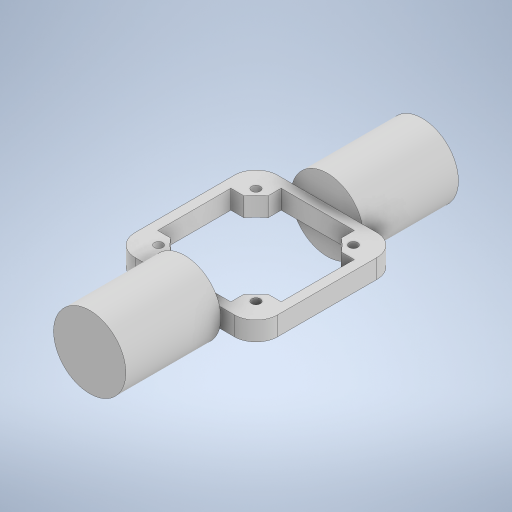
# Autodesk Inventor part: FrontPlateV2
Saved by Autodesk Inventor 2024 (Build 280153000, 153)
## iProperties
Created: 2024-02-08
Part Number: FrontPlateV2
Material: Generic
Document SubType Name: Modeling
Designer: yusuf
Density: 1 g/cm^3
Appearance: Default
Author: yusuf
Autodesk Inventor part; units mm, degrees
ref_plane "YZ Plane" through (0, 0, 0) normal (1, 0, 0) x (0, 1, 0)
ref_plane "XZ Plane" through (0, 0, 0) normal (0, 1, 0) x (-1, 0, 0)
ref_plane "XY Plane" through (0, 0, 0) normal (0, 0, 1) x (1, 0, 0)
sketch "Sketch1" plane through (0, 0, 0) normal (0, 0, 1) x (1, 0, 0)
  circle A0 centre (0, 0) radius 38
  dimension "d0" = 76
  constraints: 1 centre point, 1 coincident
  measures "d0" diameter of A0
extrude "Extrusion1" add sketch "Sketch1" along normal blind 100
sketch "Sketch2" plane through (0, 0, 0) normal (0, 0, -1) x (-1, 0, 0)
  circle A0 centre (0, 0) radius 8.75
  line L0 (0, 8.75) -> (0, 11.75)
  line L1 (0, 11.75) -> (4, 11.75)
  line L2 (4, 11.75) -> (-4, 11.75)
  line L3 (-4, 11.75) -> (-4, 7.7822)
  line L4 (4, 11.75) -> (4, 7.7822)
  dimension "d3" = 17.5
  dimension "d5" = 3
  dimension "d6" = 4
  dimension "d7" = 8
  dimension "d8" = 3.9678
  dimension "d9" = 3.9678
  constraints: 10 end point, 3 point on circle, 2 vertical, 1 centre point, 1 coincident, 1 horizontal, 1 point on line
  measures "d3" diameter of A0
  measures "d5" distance of L0.start L0.end
  measures "d6" distance of L0.end L1.end
  measures "d7" distance of L1.end L2.end
  measures "d8" distance of L2.end L3.end
  measures "d9" distance of L1.end L4.end
extrude "Extrusion2" cut sketch "Sketch2" against normal blind 90
fillet "Fillet1" radius 0.5 4 edges at (4, 9.7661, 0) (0, 11.75, 0) (-4, 9.7661, 0) (0, -8.75, 0)
fillet "Fillet2" radius 0.5 4 edges at (-4, 7.7822, 45.25) (-4.1498, 7.8731, 0.1431) (4, 7.7822, 45.25) (4.1498, 7.8731, 0.1431)
sketch "Sketch5" plane through (0, 0, 100) normal (0, 0, 1) x (1, 0, 0)
  line L0 (-75, -10) -> (75, -10)
  line L1 (75, -10) -> (75, 10)
  line L2 (75, 10) -> (-75, 10)
  line L3 (-75, 10) -> (-75, -10)
  line L4 (-75, -10) -> (75, 10) construction
  line L5 (75, -10) -> (-75, 10) construction
  point P0 (0, 0)
  dimension "d32" = 150
  dimension "d33" = 20
  constraints: 12 end point, 2 midpoint, 2 parallel, 1 horizontal, 1 perpendicular
  measures "d32" distance of L1.end L2.end
  measures "d33" distance of L0.end L1.end
extrude "Extrusion5" add sketch "Sketch5" along normal blind 150
fillet "Fillet6" radius 22.751 4 edges at (-75, 0, 250) (75, 0, 250) (75, 0, 100) (-75, 0, 100)
sketch "Sketch8" plane through (0, 0, 250) normal (0, 0, 1) x (1, 0, 0)
  circle A0 centre (0, 0) radius 38
  constraints: 1 centre point, 1 coincident
extrude "Extrusion8" add sketch "Sketch8" along normal blind 100
sketch "Sketch11" plane through (-36.6606, 10, 100) normal (0, 1, 0) x (1, 0, 0)
  line L0 (-28.3394, -140) -> (101.6606, -140)
  line L1 (101.6606, -140) -> (101.6606, -10)
  line L2 (101.6606, -10) -> (-28.3394, -10)
  line L3 (-28.3394, -10) -> (-28.3394, -140)
  line L4 (-28.3394, -140) -> (101.6606, -10) construction
  line L5 (101.6606, -140) -> (-28.3394, -10) construction
  line L6 (-38.3394, -22.751) -> (-38.3394, -127.249) projected
  line L7 (0, -150) -> (73.3212, -150) projected
  line L8 (-38.3394, -127.249) -> (-28.3394, -127.249)
  line L9 (-15.5884, -150) -> (0, -150) projected
  line L10 (-15.5884, -150) -> (-15.5884, -140)
  line L11 (-38.3394, -22.751) -> (-38.3394, -127.249) projected
  line L12 (-38.3394, -22.751) -> (-28.3394, -22.751)
  arc A0 (-15.5884, 0) -> (-38.3394, -22.751) centre (-15.5884, -22.751) ccw projected
  line L13 (-15.5884, 0) -> (-15.5884, -10)
  line L14 (88.9096, 0) -> (73.3212, 0) projected
  line L15 (88.9096, 0) -> (88.9096, -10)
  arc A1 (111.6606, -22.751) -> (88.9096, 0) centre (88.9096, -22.751) ccw projected
  line L16 (111.6606, -22.751) -> (101.6606, -22.751)
  line L17 (73.3212, -150) -> (88.9096, -150) projected
  line L18 (88.9096, -150) -> (88.9096, -140)
  line L19 (111.6606, -22.751) -> (111.6606, -127.249) projected
  line L20 (111.6606, -127.249) -> (101.6606, -127.249)
  line L21 (-28.3394, -75) -> (-28.3394, -36.5)
  line L22 (-28.3394, -75) -> (-28.3394, -113.5)
  line L23 (-28.3394, -36.5) -> (-14.5394, -36.5)
  line L24 (36.6606, -10) -> (-1.8394, -10)
  line L25 (36.6606, -10) -> (75.1606, -10)
  line L26 (-1.8394, -10) -> (-1.8394, -23.8)
  arc A2 (-1.8394, -23.8) -> (-14.5394, -36.5) centre (36.832, -75.1714) ccw
  line L27 (36.6606, -140) -> (-1.8394, -140)
  line L28 (36.6606, -140) -> (75.1606, -140)
  line L29 (101.6606, -75) -> (101.6606, -113.5)
  line L30 (101.6606, -75) -> (101.6606, -36.5)
  line L31 (36.6606, -10) -> (75.1606, -10)
  line L32 (-28.3394, -113.5) -> (-14.5394, -113.5)
  line L33 (-1.8394, -140) -> (-1.8394, -126.2)
  line L34 (75.1606, -140) -> (75.1606, -126.2)
  line L35 (101.6606, -113.5) -> (87.8606, -113.5)
  line L36 (101.6606, -36.5) -> (87.8606, -36.5)
  line L37 (75.1606, -10) -> (75.1606, -23.8)
  arc A3 (75.1606, -126.2) -> (87.8606, -113.5) centre (36.4892, -74.8286) ccw
  arc A4 (-14.5394, -113.5) -> (-1.8394, -126.2) centre (36.832, -74.8286) ccw
  arc A5 (87.8606, -36.5) -> (75.1606, -23.8) centre (36.4892, -75.1714) ccw
  point P0 (36.6606, 100)
  point P1 (36.6606, -75)
  dimension "d72" = 130
  dimension "d73" = 130
  dimension "d74" = 75
  dimension "d75" = 75
  dimension "d84" = 38.5
  dimension "d85" = 38.5
  dimension "d86" = 13.8
  dimension "d87" = 38.5
  dimension "d88" = 38.5
  dimension "d89" = 13.8
  dimension "d90" = 64.3
  dimension "d96" = 38.5
  dimension "d97" = 38.5
  dimension "d98" = 38.5
  dimension "d99" = 38.5
  dimension "d100" = 13.8
  dimension "d101" = 13.8
  dimension "d102" = 13.8
  dimension "d103" = 13.8
  dimension "d104" = 13.8
  dimension "d105" = 13.8
  dimension "d106" = 64.3
  dimension "d107" = 64.3
  dimension "d108" = 64.3
  constraints: 62 end point, 20 point on line, 8 point on circle, 6 midpoint, 5 horizontal, 5 perpendicular, 4 centre point, 4 vertical, 3 equal length
  measures "d72" distance of L1.end L2.end
  measures "d73" distance of L0.end L1.end
  measures "d74" distance from line of point (36.661, -75) L6
  measures "d75" distance from line of L7 point (36.661, -75)
  measures "d84" distance of L21.start L21.end
  measures "d85" distance of L21.start L22.end
  measures "d86" distance of L21.end L23.end
  measures "d87" distance of L24.start L24.end
  measures "d88" distance of L24.start L25.end
  measures "d89" distance of L24.end L26.end
  measures "d90" radius of A2
  measures "d96" distance of L27.start L27.end
  measures "d97" distance of L27.start L28.end
  measures "d98" distance of L29.start L29.end
  measures "d99" distance of L29.start L30.end
  measures "d100" distance of L22.end L32.end
  measures "d101" distance of L27.end L33.end
  measures "d102" distance of L28.end L34.end
  measures "d103" distance of L29.end L35.end
  measures "d104" distance of L30.end L36.end
  measures "d105" distance of L25.end L37.end
  measures "d106" radius of A3
  measures "d107" radius of A4
  measures "d108" radius of A5
extrude "Extrusion10" cut sketch "Sketch11" against normal blind 20 contours L33 A4 L32 L3 L23 A2 L26 L2 L37 A5 L36 L1 L35 A3 L34 L0
sketch "Sketch12" plane through (-36.6606, 10, 100) normal (0, 1, 0) x (1, 0, 0)
  circle A0 centre (-14.6044, -23.735) radius 4.5
  line L0 (-28.3394, -36.5) -> (-14.5394, -36.5) projected
  line L1 (-28.3394, -113.5) -> (-28.3394, -36.5) projected
  circle A1 centre (-14.6044, -126.265) radius 4.5
  circle A2 centre (87.9256, -126.265) radius 4.5
  circle A3 centre (87.9256, -23.735) radius 4.5
  line L2 (-14.5394, -113.5) -> (-28.3394, -113.5) projected
  line L3 (101.6606, -113.5) -> (87.8606, -113.5) projected
  line L4 (101.6606, -36.5) -> (101.6606, -113.5) projected
  line L5 (87.8606, -36.5) -> (101.6606, -36.5) projected
  point P0 (36.6606, 100)
  point P1 (-28.3394, -127.249)
  dimension "d91" = 9
  dimension "d92" = 12.765
  dimension "d93" = 13.735
  dimension "d109" = 9
  dimension "d110" = 9
  dimension "d111" = 9
  dimension "d112" = 12.765
  dimension "d113" = 13.735
  dimension "d114" = 12.765
  dimension "d115" = 13.735
  dimension "d116" = 13.735
  dimension "d117" = 12.765
  constraints: 4 centre point
  measures "d91" diameter of A0
  measures "d92" distance from line of A0.centre L0
  measures "d93" distance from line of L1 A0.centre
  measures "d109" diameter of A1
  measures "d110" diameter of A2
  measures "d111" diameter of A3
  measures "d112" distance from line of L2 A1.centre
  measures "d113" distance from line of L1 A1.centre
  measures "d114" distance from line of L3 A2.centre
  measures "d115" distance from line of L4 A2.centre
  measures "d116" distance from line of L4 A3.centre
  measures "d117" distance from line of L5 A3.centre
extrude "Extrusion11" cut sketch "Sketch12" against normal blind 20
equation "\"d112\" = d92"
equation "\"d113\" = d93"
equation "\"d114\" = d112"
equation "\"d115\" = d113"
equation "\"d116\" = d115"
equation "\"d117\" = d114"
body "Solid1"
